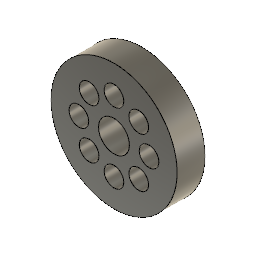
tut 1_P6 (Autodesk Fusion 360 design; units mm, degrees)
Autodesk Fusion 360 part; units mm, degrees
note: some values were not read from the file. Chosen so that the rebuilt part matches the saved one: which face or edge a step refers to.
sketch "Sketch1" plane through (0, 0, 0) normal (0, 1, 0) x (1, 0, 0)
  circle A0 centre (0, 0) radius 11
  circle A1 centre (0, 0) radius 45
  circle A2 centre (0, -25) radius 7
  dimension "d1" = 22
  dimension "d2" = 14
  measures "d1" diameter of A0
  measures "d2" diameter of A2
extrude "Extrude1" add sketch "Sketch1" along normal mid plane 20
pattern_circular "C-Pattern1" count 8 over 360 about axis through (0, 1.75, 0) along (0, 1, 0) of 2 faces at (6.9094, 6.6667, 26.1229) (6.9094, -6.6667, 26.1229)
